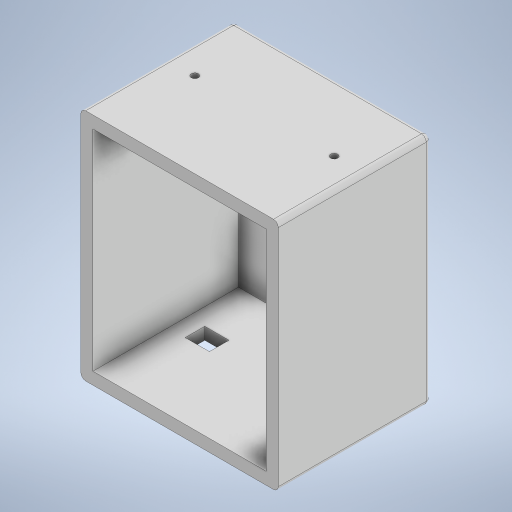
# Autodesk Inventor part: Component_shild_layered_TOPHAT
Saved by Autodesk Inventor 2024 (Build 280153000, 153)
## iProperties
Created: 2024-10-22
Part Number: Component_shild_layered_TOPHAT
Material: Generic
Document SubType Name: Modeling
Designer: Bruger
Density: 1 g/cm^3
Appearance: Default
Author: Bruger
Autodesk Inventor part; units mm, degrees
ref_plane "YZ Plane" through (0, 0, 0) normal (1, 0, 0) x (0, 1, 0)
ref_plane "XZ Plane" through (0, 0, 0) normal (0, 1, 0) x (-1, 0, 0)
ref_plane "XY Plane" through (0, 0, 0) normal (0, 0, 1) x (1, 0, 0)
sketch "Sketch1" plane through (0, 0, 0) normal (0, 0, 1) x (1, 0, 0)
  line L0 (0, 0) -> (81.43, 0)
  line L1 (81.43, 0) -> (81.43, 96.5)
  line L2 (81.43, 96.5) -> (0, 96.5)
  line L3 (0, 96.5) -> (0, 0)
  line L4 (5, 91.5) -> (76.43, 91.5)
  line L5 (76.43, 91.5) -> (76.43, 5)
  line L6 (76.43, 5) -> (5, 5)
  line L7 (5, 5) -> (5, 91.5)
  dimension "d1" = 81.43
  dimension "d2" = 96.5
  dimension "d3" = 5
  dimension "d4" = 5
  dimension "d5" = 5
  dimension "d6" = 5
  constraints: 16 end point, 4 parallel, 2 horizontal, 2 perpendicular
  measures "d1" distance between parallel lines of L1 L3
  measures "d2" distance between parallel lines of L0 L2
  measures "d3" distance between parallel lines of L7 L3
  measures "d4" distance between parallel lines of L1 L5
  measures "d5" distance between parallel lines of L4 L2
  measures "d6" distance between parallel lines of L0 L6
extrude "Extrusion1" add sketch "Sketch1" against normal blind 3 contours L3 L2 L1 L0 | L4 L5 L6 L7
extrude "Extrusion2" add sketch "Sketch1" along normal blind 60
fillet "Fillet5" radius 2 2 edges at (0, 48.25, -3) (81.43, 48.25, -3)
fillet "Fillet6" radius 2 10 edges at (0.5858, 0, -2.4142) (0, 0, 29.5) (80.8442, 0, -2.4142) (81.43, 0, 29.5) (40.715, 0, -3) (80.8442, 96.5, -2.4142) (81.43, 96.5, 29.5) (0.5858, 96.5, -2.4142) (0, 96.5, 29.5) (40.715, 96.5, -3)
sketch "Sketch3" plane through (2, 0, 60) normal (0, -1, 0) x (1, 0, 0)
  line L0 (77.43, 0) -> (0, 0)
  line L1 (67.43, -39.1) -> (57.43, -39.1)
  line L2 (57.43, -39.1) -> (57.43, -31)
  line L3 (57.43, -31) -> (67.43, -31)
  line L4 (67.43, -31) -> (67.43, -39.1)
  line L5 (77.43, 0) -> (77.43, -61) projected
  line L6 (77.43, -61) -> (0, -61) projected
  line L7 (20, -31) -> (10, -31)
  line L8 (10, -31) -> (10, -39.1)
  line L9 (10, -39.1) -> (20, -39.1)
  line L10 (20, -39.1) -> (20, -31)
  line L11 (0, -61) -> (0, 0) projected
  point P0 (-2, -60)
  point P1 (77.43, -30)
  point P2 (76.43, -31)
  point P3 (1, -31)
  point P4 (0, -30)
  point P5 (10, -35.05)
  point P6 (73.8173, -31)
  point P7 (3.6124, -31)
  dimension "d38" = 10
  dimension "d39" = 8.1
  dimension "d40" = 10
  dimension "d41" = 21.9
  dimension "d42" = 10
  dimension "d43" = 8.1
  dimension "d44" = 21.9
  dimension "d45" = 10
  constraints: 18 end point, 4 parallel, 3 horizontal, 2 perpendicular, 1 midpoint, 1 other
  measures "d38" distance of L1.start L1.end
  measures "d39" distance of L1.end L2.end
  measures "d40" distance between parallel lines of L5 L4
  measures "d42" distance of L8.end L9.end
  measures "d43" distance of L7.end L8.end
  measures "d45" distance from line of L11 point (10, -35.05)
extrude "Extrusion3" cut sketch "Sketch3" against normal blind 5 contours L1 L2 L3 L4 | L10 L9 L8 L7
sketch "Sketch4" plane through (2, 96.5, 60) normal (0, 1, 0) x (1, 0, 0)
  circle A0 centre (10, 35) radius 4
  line L0 (0, 61) -> (77.43, 61) projected
  line L1 (0, 0) -> (0, 61) projected
  circle A1 centre (67.43, 35) radius 4
  line L2 (77.43, 61) -> (77.43, 0) projected
  point P0 (-2, 60)
  point P1 (1, 31)
  point P2 (76.43, 31)
  point P3 (0, 30)
  point P4 (77.43, 30)
  point P5 (3.6123, 31)
  point P6 (73.8174, 31)
  dimension "d48" = 8
  dimension "d49" = 26
  dimension "d50" = 10
  dimension "d51" = 8
  dimension "d52" = 26
  dimension "d53" = 10
  constraints: 2 centre point, 1 other
  measures "d48" diameter of A0
  measures "d50" distance from line of L1 A0.centre
  measures "d51" diameter of A1
  measures "d53" distance from line of L2 A1.centre
hole "Hole2" at (69.43, 96.5, 25) at (12, 96.5, 25) direction (0, -1, 0) diameter 2.95 depth 5 tip angle 118
equation "\"d52\" = d49"
body "Solid1"
